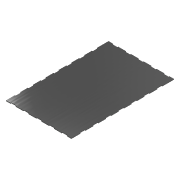
# Autodesk Inventor part: base inferior
Saved by Autodesk Inventor 2020 (Build 240168000, 168)
## iProperties
Created: 2021-09-21
Part Number: base inferior
Material: Generic
Document SubType Name: Modeling
Designer: pablo
Density: 1 g/cm^3
Appearance: Dark Gray
Author: pablo
Autodesk Inventor part; units mm, degrees
ref_plane "YZ Plane" through (0, 0, 0) normal (1, 0, 0) x (0, 1, 0)
ref_plane "XZ Plane" through (0, 0, 0) normal (0, 1, 0) x (-1, 0, 0)
ref_plane "XY Plane" through (0, 0, 0) normal (0, 0, 1) x (1, 0, 0)
sketch "Sketch1" plane through (0, 0, 0) normal (0, 1, 0) x (-1, 0, 0)
  line L0 (127.5, -200) -> (-127.5, -200)
  line L1 (-127.5, -200) -> (-127.5, 200)
  line L2 (-127.5, 200) -> (127.5, 200)
  line L3 (127.5, 200) -> (127.5, -200)
  line L4 (127.5, -200) -> (-127.5, 200) construction
  line L5 (-127.5, -200) -> (127.5, 200) construction
  point P0 (0, 0)
  dimension "d0" = 255
  dimension "d1" = 400
  constraints: 12 end point, 2 midpoint, 2 parallel, 1 horizontal, 1 perpendicular
  measures "d0" distance of L1.end L2.end
  measures "d1" distance of L0.end L1.end
extrude "base" add sketch "Sketch1" along normal blind 3
sketch "Sketch5" plane through (0, 3, 0) normal (0, 1, 0) x (1, 0, 0)
  line L0 (-127.5, -200) -> (127.5, -200) projected
  line L1 (-110, -200) -> (-90, -200)
  line L2 (-90, -200) -> (-90, -197)
  line L3 (-90, -197) -> (-110, -197)
  line L4 (-110, -197) -> (-110, -200)
  line L5 (-60, -200) -> (-40, -200)
  line L6 (-40, -200) -> (-40, -197)
  line L7 (-40, -197) -> (-60, -197)
  line L8 (-60, -197) -> (-60, -200)
  line L9 (-10, -200) -> (10, -200)
  line L10 (10, -200) -> (10, -197)
  line L11 (10, -197) -> (-10, -197)
  line L12 (-10, -197) -> (-10, -200)
  line L13 (40, -200) -> (60, -200)
  line L14 (60, -200) -> (60, -197)
  line L15 (60, -197) -> (40, -197)
  line L16 (40, -197) -> (40, -200)
  line L17 (90, -200) -> (110, -200)
  line L18 (110, -200) -> (110, -197)
  line L19 (110, -197) -> (90, -197)
  line L20 (90, -197) -> (90, -200)
  line L21 (-110, 200) -> (-110, 197)
  line L22 (-90, 200) -> (-110, 200)
  line L23 (-110, 197) -> (-90, 197)
  line L24 (-90, 197) -> (-90, 200)
  line L25 (-60, 200) -> (-60, 197)
  line L26 (-40, 200) -> (-60, 200)
  line L27 (-40, 197) -> (-40, 200)
  line L28 (-10, 200) -> (-10, 197)
  line L29 (10, 200) -> (-10, 200)
  line L30 (10, 197) -> (10, 200)
  line L31 (-10, 197) -> (10, 197)
  line L32 (-60, 197) -> (-40, 197)
  line L33 (40, 200) -> (40, 197)
  line L34 (40, 197) -> (60, 197)
  line L35 (60, 200) -> (40, 200)
  line L36 (60, 197) -> (60, 200)
  line L37 (90, 200) -> (90, 197)
  line L38 (90, 197) -> (110, 197)
  line L39 (110, 200) -> (90, 200)
  line L40 (110, 197) -> (110, 200)
  point P0 (0, 0)
  point P1 (90, -200)
  point P2 (110, -200)
  point P3 (-10, -200)
  point P4 (10, -200)
  point P5 (-60, -200)
  point P6 (-40, -200)
  point P7 (40, -200)
  point P8 (60, -200)
  dimension "d36" = 20
  dimension "d37" = 3
  dimension "d40" = 50
  dimension "d45" = 17.5
  dimension "d46" = 17.5
  dimension "d49" = 397
  constraints: 80 end point, 2 horizontal, 2 parallel, 1 collinear, 1 perpendicular, 1 point on line, 1 vertical, 71 other
  measures "d36" distance of L3.end L2.end
  measures "d37" distance of L2.end L1.end
  measures "d40" distance of L1.start L5.start
  measures "d45" distance of L0.start L1.start
  measures "d46" distance of L17.end L0.end
  measures "d49" distance of L1.start L21.end
extrude "Extrusion4" cut sketch "Sketch5" against normal blind 5
sketch "Sketch8" plane through (0, 3, 0) normal (0, 1, 0) x (1, 0, 0)
  line L0 (-127.5, 200) -> (-127.5, -200) projected
  line L1 (-127.5, -145) -> (-124.5, -145)
  line L2 (-124.5, -145) -> (-124.5, -165)
  line L3 (-124.5, -165) -> (-127.5, -165)
  line L4 (-127.5, -165) -> (-127.5, -145)
  line L5 (-127.5, -95) -> (-124.5, -95)
  line L6 (-124.5, -95) -> (-124.5, -115)
  line L7 (-124.5, -115) -> (-127.5, -115)
  line L8 (-127.5, -115) -> (-127.5, -95)
  line L9 (-127.5, -45) -> (-124.5, -45)
  line L10 (-124.5, -45) -> (-124.5, -65)
  line L11 (-124.5, -65) -> (-127.5, -65)
  line L12 (-127.5, -65) -> (-127.5, -45)
  line L13 (-127.5, 5) -> (-124.5, 5)
  line L14 (-124.5, 5) -> (-124.5, -15)
  line L15 (-124.5, -15) -> (-127.5, -15)
  line L16 (-127.5, -15) -> (-127.5, 5)
  line L17 (-127.5, 55) -> (-124.5, 55)
  line L18 (-124.5, 55) -> (-124.5, 35)
  line L19 (-124.5, 35) -> (-127.5, 35)
  line L20 (-127.5, 35) -> (-127.5, 55)
  line L21 (-127.5, 105) -> (-124.5, 105)
  line L22 (-124.5, 105) -> (-124.5, 85)
  line L23 (-124.5, 85) -> (-127.5, 85)
  line L24 (-127.5, 85) -> (-127.5, 105)
  line L25 (-127.5, 155) -> (-124.5, 155)
  line L26 (-124.5, 155) -> (-124.5, 135)
  line L27 (-124.5, 135) -> (-127.5, 135)
  line L28 (-127.5, 135) -> (-127.5, 155)
  line L29 (0, 0) -> (0, -33.5633)
  line L30 (127.5, -145) -> (124.5, -145)
  line L31 (124.5, -145) -> (124.5, -165)
  line L32 (124.5, -165) -> (127.5, -165)
  line L33 (127.5, -165) -> (127.5, -145)
  line L34 (127.5, -95) -> (124.5, -95)
  line L35 (124.5, -95) -> (124.5, -115)
  line L36 (124.5, -115) -> (127.5, -115)
  line L37 (127.5, -115) -> (127.5, -95)
  line L38 (127.5, -45) -> (124.5, -45)
  line L39 (124.5, -45) -> (124.5, -65)
  line L40 (124.5, -65) -> (127.5, -65)
  line L41 (127.5, -65) -> (127.5, -45)
  line L42 (127.5, 5) -> (124.5, 5)
  line L43 (124.5, 5) -> (124.5, -15)
  line L44 (124.5, -15) -> (127.5, -15)
  line L45 (127.5, -15) -> (127.5, 5)
  line L46 (127.5, 55) -> (124.5, 55)
  line L47 (124.5, 55) -> (124.5, 35)
  line L48 (124.5, 35) -> (127.5, 35)
  line L49 (127.5, 35) -> (127.5, 55)
  line L50 (127.5, 105) -> (124.5, 105)
  line L51 (124.5, 105) -> (124.5, 85)
  line L52 (124.5, 85) -> (127.5, 85)
  line L53 (127.5, 85) -> (127.5, 105)
  line L54 (127.5, 155) -> (124.5, 155)
  line L55 (124.5, 155) -> (124.5, 135)
  line L56 (124.5, 135) -> (127.5, 135)
  line L57 (127.5, 135) -> (127.5, 155)
  dimension "d82" = 3
  dimension "d83" = 20
  dimension "d84" = 35
  dimension "d87" = 50
  constraints: 114 end point, 28 symmetric about line, 2 parallel, 2 vertical, 1 horizontal, 1 perpendicular, 1 point on line, 48 other
  measures "d82" distance of L2.end L3.end
  measures "d83" distance of L1.end L2.end
  measures "d84" distance of L3.end L0.end
  measures "d87" distance of L1.start L5.start
extrude "Extrusion7" cut sketch "Sketch8" against normal blind 5
body "Solid1"
